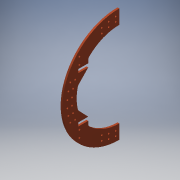
# Autodesk Inventor part: 16in inner coil
Saved by Autodesk Inventor 2016 (Build 200138000, 138)
## iProperties
Created: 2016-01-31
Part Number: 16in inner coil
Material: Copper
Document SubType Name: Modeling
Designer: Scott
Density: 8.94 g/cm^3
Appearance: Copper - Satin
Author: Scott
Autodesk Inventor part; units mm, degrees
ref_plane "YZ Plane" through (0, 0, 0) normal (1, 0, 0) x (0, 1, 0)
ref_plane "XZ Plane" through (0, 0, 0) normal (0, 1, 0) x (-1, 0, 0)
ref_plane "XY Plane" through (0, 0, 0) normal (0, 0, 1) x (1, 0, 0)
sketch "Sketch1" plane through (0, 0, 0) normal (1, 0, 0) x (0, 1, 0)
  arc A0 (203.2, 0) -> (-203.2, 0) centre (0, 0) ccw
  arc A1 (152.4, 0) -> (-152.4, 0) centre (0, 0) ccw
  arc A2 (185.42, 0) -> (-185.42, 0) centre (0, 0) ccw
  line L0 (0, 0) -> (152.4, 0) construction
  line L1 (0, 0) -> (220.2471, 220.2471) construction
  line L2 (0, 0) -> (-217.8171, 217.8171) construction
  line L3 (0, 0) -> (-152.4, 0) construction
  line L4 (203.2, 0) -> (418.8667, 0) construction
  line L5 (152.4, 0) -> (-185.42, 0)
  line L6 (-203.2, 0) -> (-272.3039, 0)
  line L7 (-185.42, 0) -> (-203.2, 0)
  line L8 (-152.4, 0) -> (-203.2, 0)
  line L9 (152.4, 0) -> (203.2, 0)
  arc A3 (168.91, 0) -> (-168.91, 0) centre (0, 0) ccw
  point P0 (181.5133, 37.8617)
  point P1 (184.9846, 12.7)
  point P2 (164.6231, 37.8128)
  point P3 (168.4319, 12.7)
  point P4 (174.6359, 62.3129)
  point P5 (157.0918, 62.0706)
  point P6 (37.8617, 181.5133)
  point P7 (12.7, 184.9846)
  point P8 (37.8128, 164.6231)
  point P9 (12.7, 168.4319)
  point P10 (62.3129, 174.6359)
  point P11 (62.0706, 157.0918)
  point P12 (-62.3129, 174.6359)
  point P13 (-37.8617, 181.5133)
  point P14 (-62.0706, 157.0918)
  point P15 (-37.8128, 164.6231)
  point P16 (-12.7, 168.4319)
  point P17 (-12.7, 184.9846)
  point P18 (-157.0918, 62.0706)
  point P19 (-174.6359, 62.3129)
  point P20 (-181.5133, 37.8617)
  point P21 (-164.6231, 37.8128)
  point P22 (-168.4319, 12.7)
  point P23 (-184.9846, 12.7)
  dimension "d0" = 406.4
  dimension "d2" = 304.8
  dimension "d3" = 370.84
  dimension "d5" = 50.8
  dimension "d6" = 25.4
  dimension "d7" = 25.4
  dimension "d8" = 12.7
  dimension "d9" = 12.7
  dimension "d10" = 25.4
  dimension "d11" = 25.4
  dimension "d12" = 45
  dimension "d13" = 45
  constraints: 20 end point, 16 point on circle, 12 symmetric about line, 4 centre point, 4 coincident, 3 horizontal, 3 point on line, 1 collinear
  measures "d0" diameter of A0
  measures "d2" diameter of A1
  measures "d3" diameter of A2
  measures "d5" radial gap between concentric circles of A1 A0
  measures "d6" distance of point (184.985, 12.7) point (181.513, 37.862)
  measures "d7" distance of point (168.432, 12.7) point (164.623, 37.813)
  measures "d8" distance from line of L0 point (184.985, 12.7)
  measures "d9" distance from line of L0 point (168.432, 12.7)
  measures "d10" distance of point (181.513, 37.862) point (174.636, 62.313)
  measures "d11" distance of point (164.623, 37.813) point (157.092, 62.071)
  measures "d12" angle of L3 L2
  measures "d13" angle of L0 L1
extrude "Extrusion1" add sketch "Sketch1" along normal blind 6.35 contours L9 A2 L7 A0 | L9 A3 L5 A2 | L9 A1 L5 A3
hole "Hole1" at (0, 181.5133, 37.8617) at (0, 184.9846, 12.7) at (0, 164.6231, 37.8128) at (0, 168.4319, 12.7) at (0, 174.6359, 62.3129) at (0, 157.0918, 62.0706) at (0, 62.3129, 174.6359) at (0, 37.8617, 181.5133) at (0, 62.0706, 157.0918) at (0, 37.8128, 164.6231) at (0, 12.7, 168.4319) at (0, 12.7, 184.9846) at (0, -62.0706, 157.0918) at (0, -62.3129, 174.6359) at (0, -37.8617, 181.5133) at (0, -37.8128, 164.6231) at (0, -12.7, 168.4319) at (0, -12.7, 184.9846) at (0, -184.9846, 12.7) at (0, -168.4319, 12.7) at (0, -181.5133, 37.8617) at (0, -164.6231, 37.8128) at (0, -174.6359, 62.3129) at (0, -157.0918, 62.0706) direction (1, 0, 0) diameter 6.604 end through all
sketch "Sketch4" plane through (0, 0, 0) normal (-1, 0, 0) x (0, 0, 1)
  line L0 (127, 92.2547) -> (157.48, 92.2547) projected
  line L1 (157.48, 150.1234) -> (157.48, 92.2547) projected
  line L2 (143.2518, 198.5102) -> (157.48, 150.1234) projected
  arc A0 (143.2518, 198.5102) -> (131.3752, 213.4606) centre (118.8834, 191.3446) ccw projected
  line L3 (127, 215.9318) -> (131.3752, 213.4606) projected
  line L4 (127, 92.2547) -> (127, 215.9318) projected
  circle A1 centre (142.24, 125.6507) radius 3.302 projected
  circle A2 centre (142.24, 100.2507) radius 3.302 projected
  circle A3 centre (142.24, -100.2507) radius 3.302 projected
  circle A4 centre (-142.24, -100.2507) radius 3.302 projected
  circle A5 centre (-142.24, -125.6507) radius 3.302 projected
  circle A6 centre (142.24, -125.6507) radius 3.302 projected
  line L5 (114.3, -183.162) -> (127, -183.162) projected
  line L6 (127, -183.162) -> (163.2323, -141.3083) projected
  arc A7 (163.2323, -141.3083) -> (215.9, 0) centre (0, 0) ccw projected
  line L7 (152.4, 0) -> (215.9, 0) projected
  arc A8 (-152.4, 0) -> (152.4, 0) centre (0, 0) ccw projected
  line L8 (-215.9, 0) -> (-152.4, 0) projected
  arc A9 (-215.9, 0) -> (-163.2323, -141.3083) centre (0, 0) ccw projected
  line L9 (-163.2323, -141.3083) -> (-127, -183.162) projected
  line L10 (-127, -183.162) -> (-114.3, -183.162) projected
  line L11 (-114.3, -183.162) -> (-114.3, -195.862) projected
  line L12 (-114.3, -195.862) -> (-46.5518, -210.8216) projected
  arc A10 (-46.5518, -210.8216) -> (46.5518, -210.8216) centre (0, 0) ccw projected
  line L13 (46.5518, -210.8216) -> (114.3, -195.862) projected
  line L14 (114.3, -195.862) -> (114.3, -183.162) projected
  circle A11 centre (174.6359, -62.3129) radius 3.302 projected
  circle A12 centre (181.5133, -37.8617) radius 3.302 projected
  circle A13 centre (184.9846, -12.7) radius 3.302 projected
  circle A14 centre (12.7, -168.4319) radius 3.302 projected
  circle A15 centre (37.8617, -181.5133) radius 3.302 projected
  circle A16 centre (62.0706, -157.0918) radius 3.302 projected
  circle A17 centre (-12.7, -168.4319) radius 3.302 projected
  circle A18 centre (-62.0706, -157.0918) radius 3.302 projected
  circle A19 centre (-62.3129, -174.6359) radius 3.302 projected
  circle A20 centre (-174.6359, -62.3129) radius 3.302 projected
  circle A21 centre (-164.6231, -37.8128) radius 3.302 projected
  circle A22 centre (-181.5133, -37.8617) radius 3.302 projected
  circle A23 centre (-184.9846, -12.7) radius 3.302 projected
  circle A24 centre (-168.4319, -12.7) radius 3.302 projected
  circle A25 centre (-157.0918, -62.0706) radius 3.302 projected
  circle A26 centre (-37.8617, -181.5133) radius 3.302 projected
  circle A27 centre (-37.8128, -164.6231) radius 3.302 projected
  circle A28 centre (-12.7, -184.9846) radius 3.302 projected
  circle A29 centre (62.3129, -174.6359) radius 3.302 projected
  circle A30 centre (37.8128, -164.6231) radius 3.302 projected
  circle A31 centre (12.7, -184.9846) radius 3.302 projected
  circle A32 centre (168.4319, -12.7) radius 3.302 projected
  circle A33 centre (164.6231, -37.8128) radius 3.302 projected
  circle A34 centre (157.0918, -62.0706) radius 3.302 projected
  point P0 (0, 0)
  constraints: 4 coincident
hole "Hole4" at (0, -125.6507, 142.24) at (0, -100.2507, 142.24) at (0, 100.2507, 142.24) at (0, 125.6507, 142.24) direction (1, 0, 0) diameter 6.604 end through all
sketch "Sketch5" plane through (0, 0, 0) normal (-1, 0, 0) x (0, 0, 1)
  line L0 (-145.9119, -88.9) -> (-106.6761, -88.9)
  line L1 (-106.6761, -88.9) -> (-106.6761, -76.2)
  line L2 (-106.6761, -76.2) -> (-145.9119, -76.2)
  line L3 (-145.9119, -76.2) -> (-145.9119, -88.9)
  line L4 (145.9119, -88.9) -> (99.5479, -88.9)
  line L5 (99.5479, -88.9) -> (99.5479, -76.2)
  line L6 (99.5479, -76.2) -> (145.9119, -76.2)
  line L7 (145.9119, -76.2) -> (145.9119, -88.9)
  line L8 (145.9119, 88.9) -> (145.9119, 76.2) projected
  line L9 (145.9119, 76.2) -> (108.0536, 76.2)
  line L10 (108.0536, 76.2) -> (108.0536, 88.9)
  line L11 (108.0536, 88.9) -> (145.9119, 88.9)
  line L12 (145.9119, 88.9) -> (145.9119, 76.2)
  point P0 (0, 0)
  constraints: 24 end point, 6 parallel, 3 horizontal, 3 perpendicular, 1 point on line
extrude "Extrusion3" cut sketch "Sketch5" against normal blind 25.4 contours L4 L5 L6 L7 | L8 L9 L10 L11
sketch "Sketch6" plane through (6.35, 0, 0) normal (1, 0, 0) x (0, 0, -1)
  circle A0 centre (-157.0918, 62.0706) radius 3.302 projected
  circle A1 centre (-164.6231, 37.8128) radius 3.302 projected
  circle A2 centre (-168.4319, 12.7) radius 3.302 projected
  circle A3 centre (-12.7, 184.9846) radius 3.302 projected
  circle A4 centre (-37.8128, 164.6231) radius 3.302 projected
  circle A5 centre (-62.3129, 174.6359) radius 3.302 projected
  circle A6 centre (12.7, 184.9846) radius 3.302 projected
  circle A7 centre (37.8128, 164.6231) radius 3.302 projected
  circle A8 centre (37.8617, 181.5133) radius 3.302 projected
  circle A9 centre (157.0918, 62.0706) radius 3.302 projected
  circle A10 centre (168.4319, 12.7) radius 3.302 projected
  circle A11 centre (184.9846, 12.7) radius 3.302 projected
  circle A12 centre (181.5133, 37.8617) radius 3.302 projected
  circle A13 centre (164.6231, 37.8128) radius 3.302 projected
  circle A14 centre (174.6359, 62.3129) radius 3.302 projected
  circle A15 centre (62.3129, 174.6359) radius 3.302 projected
  circle A16 centre (62.0706, 157.0918) radius 3.302 projected
  circle A17 centre (12.7, 168.4319) radius 3.302 projected
  circle A18 centre (-62.0706, 157.0918) radius 3.302 projected
  circle A19 centre (-37.8617, 181.5133) radius 3.302 projected
  circle A20 centre (-12.7, 168.4319) radius 3.302 projected
  circle A21 centre (-184.9846, 12.7) radius 3.302 projected
  circle A22 centre (-181.5133, 37.8617) radius 3.302 projected
  circle A23 centre (-174.6359, 62.3129) radius 3.302 projected
  line L0 (-123.8289, 76.2) -> (-145.9119, 76.2) projected
  line L1 (-145.9119, 76.2) -> (-145.9119, 88.9) projected
  line L2 (-145.9119, 88.9) -> (-123.7843, 88.9) projected
  arc A24 (123.7843, 88.9) -> (-123.7843, 88.9) centre (0, 0) ccw projected
  line L3 (123.7843, 88.9) -> (145.9119, 88.9) projected
  line L4 (145.9119, 88.9) -> (145.9119, 76.2) projected
  line L5 (145.9119, 76.2) -> (123.825, 76.2) projected
  line L6 (123.825, 76.2) -> (147.5607, 38.1) projected
  arc A25 (152.4, 0) -> (147.5607, 38.1) centre (0, 0) ccw projected
  line L7 (215.9, 0) -> (152.4, 0) projected
  arc A26 (215.9, 0) -> (163.2323, 141.3083) centre (0, 0) ccw projected
  line L8 (163.2323, 141.3083) -> (127, 183.162) projected
  line L9 (127, 183.162) -> (114.3, 183.162) projected
  line L10 (114.3, 183.162) -> (114.3, 195.862) projected
  line L11 (114.3, 195.862) -> (46.5518, 210.8216) projected
  arc A27 (46.5518, 210.8216) -> (-46.5518, 210.8216) centre (0, 0) ccw projected
  line L12 (-46.5518, 210.8216) -> (-114.3, 195.862) projected
  line L13 (-114.3, 195.862) -> (-114.3, 183.162) projected
  line L14 (-114.3, 183.162) -> (-127, 183.162) projected
  line L15 (-127, 183.162) -> (-163.2323, 141.3083) projected
  arc A28 (-163.2323, 141.3083) -> (-215.9, 0) centre (0, 0) ccw projected
  line L16 (-152.4, 0) -> (-215.9, 0) projected
  arc A29 (-147.5607, 38.1) -> (-152.4, 0) centre (0, 0) ccw projected
  line L17 (-147.5607, 38.1) -> (-123.8289, 76.2) projected
  circle A30 centre (-142.24, 125.6507) radius 3.302 projected
  circle A31 centre (142.24, 125.6507) radius 3.302 projected
  circle A32 centre (142.24, 100.2507) radius 3.302 projected
  circle A33 centre (-142.24, 100.2507) radius 3.302 projected
  circle A34 centre (157.0918, -62.0706) radius 3.302 projected
  circle A35 centre (164.6231, -37.8128) radius 3.302 projected
  circle A36 centre (168.4319, -12.7) radius 3.302 projected
  circle A37 centre (12.7, -184.9846) radius 3.302 projected
  circle A38 centre (37.8128, -164.6231) radius 3.302 projected
  circle A39 centre (62.3129, -174.6359) radius 3.302 projected
  circle A40 centre (-12.7, -184.9846) radius 3.302 projected
  circle A41 centre (-37.8128, -164.6231) radius 3.302 projected
  circle A42 centre (-37.8617, -181.5133) radius 3.302 projected
  circle A43 centre (-157.0918, -62.0706) radius 3.302 projected
  circle A44 centre (-168.4319, -12.7) radius 3.302 projected
  circle A45 centre (-184.9846, -12.7) radius 3.302 projected
  circle A46 centre (-181.5133, -37.8617) radius 3.302 projected
  circle A47 centre (-164.6231, -37.8128) radius 3.302 projected
  circle A48 centre (-174.6359, -62.3129) radius 3.302 projected
  circle A49 centre (-62.3129, -174.6359) radius 3.302 projected
  circle A50 centre (-62.0706, -157.0918) radius 3.302 projected
  circle A51 centre (-12.7, -168.4319) radius 3.302 projected
  circle A52 centre (62.0706, -157.0918) radius 3.302 projected
  circle A53 centre (37.8617, -181.5133) radius 3.302 projected
  circle A54 centre (12.7, -168.4319) radius 3.302 projected
  circle A55 centre (184.9846, -12.7) radius 3.302 projected
  circle A56 centre (181.5133, -37.8617) radius 3.302 projected
  circle A57 centre (174.6359, -62.3129) radius 3.302 projected
  line L18 (123.8289, -76.2) -> (145.9119, -76.2) projected
  line L19 (145.9119, -76.2) -> (145.9119, -88.9) projected
  line L20 (145.9119, -88.9) -> (123.7843, -88.9) projected
  arc A58 (-123.7843, -88.9) -> (123.7843, -88.9) centre (0, 0) ccw projected
  line L21 (-123.7843, -88.9) -> (-145.9119, -88.9) projected
  line L22 (-145.9119, -88.9) -> (-145.9119, -76.2) projected
  line L23 (-145.9119, -76.2) -> (-123.825, -76.2) projected
  line L24 (-123.825, -76.2) -> (-147.5607, -38.1) projected
  arc A59 (-152.4, 0) -> (-147.5607, -38.1) centre (0, 0) ccw projected
  line L25 (-215.9, 0) -> (-152.4, 0) projected
  arc A60 (-215.9, 0) -> (-163.2323, -141.3083) centre (0, 0) ccw projected
  line L26 (-163.2323, -141.3083) -> (-127, -183.162) projected
  line L27 (-127, -183.162) -> (-114.3, -183.162) projected
  line L28 (-114.3, -183.162) -> (-114.3, -195.862) projected
  line L29 (-114.3, -195.862) -> (-46.5518, -210.8216) projected
  arc A61 (-46.5518, -210.8216) -> (46.5518, -210.8216) centre (0, 0) ccw projected
  line L30 (46.5518, -210.8216) -> (114.3, -195.862) projected
  line L31 (114.3, -195.862) -> (114.3, -183.162) projected
  line L32 (114.3, -183.162) -> (127, -183.162) projected
  line L33 (127, -183.162) -> (163.2323, -141.3083) projected
  arc A62 (163.2323, -141.3083) -> (215.9, 0) centre (0, 0) ccw projected
  line L34 (152.4, 0) -> (215.9, 0) projected
  arc A63 (147.5607, -38.1) -> (152.4, 0) centre (0, 0) ccw projected
  line L35 (147.5607, -38.1) -> (123.8289, -76.2) projected
  circle A64 centre (142.24, -125.6507) radius 3.302 projected
  circle A65 centre (-142.24, -125.6507) radius 3.302 projected
  circle A66 centre (-142.24, -100.2507) radius 3.302 projected
  circle A67 centre (142.24, -100.2507) radius 3.302 projected
  arc A68 (-131.9823, 76.2) -> (-131.9823, -76.2) centre (0, 0) ccw projected
extrude "Extrusion4" add sketch "Sketch6" against normal blind 6.35 contours L17 A68 L0 | L24 L23 A68
sketch "Sketch7" plane through (6.35, 0, 0) normal (1, 0, 0) x (0, 0, -1)
  arc A0 (152.4, 0) -> (148.406, 34.6616) centre (0, 0) ccw projected
  line L0 (215.9, 0) -> (152.4, 0) projected
  arc A1 (215.9, 0) -> (163.2323, 141.3083) centre (0, 0) ccw projected
  line L1 (163.2323, 141.3083) -> (127, 183.162) projected
  line L2 (127, 183.162) -> (114.3, 183.162) projected
  line L3 (114.3, 183.162) -> (114.3, 195.862) projected
  line L4 (114.3, 195.862) -> (46.5518, 210.8216) projected
  arc A2 (46.5518, 210.8216) -> (-46.5518, 210.8216) centre (0, 0) ccw projected
  line L5 (-46.5518, 210.8216) -> (-114.3, 195.862) projected
  line L6 (-114.3, 195.862) -> (-114.3, 183.162) projected
  line L7 (-114.3, 183.162) -> (-127, 183.162) projected
  line L8 (-127, 183.162) -> (-163.2323, 141.3083) projected
  arc A3 (-163.2323, 141.3083) -> (-215.9, 0) centre (0, 0) ccw projected
  line L9 (-152.4, 0) -> (-215.9, 0) projected
  arc A4 (-148.406, 34.6616) -> (-152.4, 0) centre (0, 0) ccw projected
  arc A5 (-145.2178, 40.5502) -> (-148.406, 34.6616) centre (-136.0388, 31.7731) ccw projected
  line L10 (-145.2178, 40.5502) -> (-111.1289, 76.2) projected
  line L11 (-111.1289, 76.2) -> (-145.9119, 76.2) projected
  line L12 (-145.9119, 76.2) -> (-145.9119, 88.9) projected
  line L13 (-145.9119, 88.9) -> (-111.0843, 88.9) projected
  line L14 (-111.0843, 88.9) -> (-111.0843, 99.1797) projected
  arc A6 (-107.3283, 108.1961) -> (-111.0843, 99.1797) centre (-98.3843, 99.1797) ccw projected
  arc A7 (107.3283, 108.1961) -> (-107.3283, 108.1961) centre (0, 0) ccw projected
  arc A8 (111.0843, 99.1797) -> (107.3283, 108.1961) centre (98.3843, 99.1797) ccw projected
  line L15 (111.0843, 88.9) -> (111.0843, 99.1797) projected
  line L16 (111.0843, 88.9) -> (145.9119, 88.9) projected
  line L17 (145.9119, 88.9) -> (145.9119, 76.2) projected
  line L18 (145.9119, 76.2) -> (111.1289, 76.2) projected
  line L19 (145.2178, 40.5502) -> (111.1289, 76.2) projected
  arc A9 (148.406, 34.6616) -> (145.2178, 40.5502) centre (136.0388, 31.7731) ccw projected
  circle A10 centre (-157.0918, 62.0706) radius 3.302 projected
  circle A11 centre (-164.6231, 37.8128) radius 3.302 projected
  circle A12 centre (-168.4319, 12.7) radius 3.302 projected
  circle A13 centre (-12.7, 184.9846) radius 3.302 projected
  circle A14 centre (-37.8128, 164.6231) radius 3.302 projected
  circle A15 centre (-62.3129, 174.6359) radius 3.302 projected
  circle A16 centre (12.7, 184.9846) radius 3.302 projected
  circle A17 centre (37.8128, 164.6231) radius 3.302 projected
  circle A18 centre (37.8617, 181.5133) radius 3.302 projected
  circle A19 centre (157.0918, 62.0706) radius 3.302 projected
  circle A20 centre (168.4319, 12.7) radius 3.302 projected
  circle A21 centre (184.9846, 12.7) radius 3.302 projected
  circle A22 centre (181.5133, 37.8617) radius 3.302 projected
  circle A23 centre (164.6231, 37.8128) radius 3.302 projected
  circle A24 centre (174.6359, 62.3129) radius 3.302 projected
  circle A25 centre (62.3129, 174.6359) radius 3.302 projected
  circle A26 centre (62.0706, 157.0918) radius 3.302 projected
  circle A27 centre (12.7, 168.4319) radius 3.302 projected
  circle A28 centre (-62.0706, 157.0918) radius 3.302 projected
  circle A29 centre (-37.8617, 181.5133) radius 3.302 projected
  circle A30 centre (-12.7, 168.4319) radius 3.302 projected
  circle A31 centre (-184.9846, 12.7) radius 3.302 projected
  circle A32 centre (-181.5133, 37.8617) radius 3.302 projected
  circle A33 centre (-174.6359, 62.3129) radius 3.302 projected
  circle A34 centre (-142.24, 125.6507) radius 3.302 projected
  circle A35 centre (142.24, 125.6507) radius 3.302 projected
  circle A36 centre (142.24, 100.2507) radius 3.302 projected
  circle A37 centre (-142.24, 100.2507) radius 3.302 projected
  arc A38 (-152.4, 0) -> (-148.406, -34.6616) centre (0, 0) ccw projected
  line L20 (-215.9, 0) -> (-152.4, 0) projected
  arc A39 (-215.9, 0) -> (-163.2323, -141.3083) centre (0, 0) ccw projected
  line L21 (-163.2323, -141.3083) -> (-127, -183.162) projected
  line L22 (-127, -183.162) -> (-114.3, -183.162) projected
  line L23 (-114.3, -183.162) -> (-114.3, -195.862) projected
  line L24 (-114.3, -195.862) -> (-46.5518, -210.8216) projected
  arc A40 (-46.5518, -210.8216) -> (46.5518, -210.8216) centre (0, 0) ccw projected
  line L25 (46.5518, -210.8216) -> (114.3, -195.862) projected
  line L26 (114.3, -195.862) -> (114.3, -183.162) projected
  line L27 (114.3, -183.162) -> (127, -183.162) projected
  line L28 (127, -183.162) -> (163.2323, -141.3083) projected
  arc A41 (163.2323, -141.3083) -> (215.9, 0) centre (0, 0) ccw projected
  line L29 (152.4, 0) -> (215.9, 0) projected
  arc A42 (148.406, -34.6616) -> (152.4, 0) centre (0, 0) ccw projected
  arc A43 (145.2178, -40.5502) -> (148.406, -34.6616) centre (136.0388, -31.7731) ccw projected
  line L30 (145.2178, -40.5502) -> (111.1289, -76.2) projected
  line L31 (111.1289, -76.2) -> (145.9119, -76.2) projected
  line L32 (145.9119, -76.2) -> (145.9119, -88.9) projected
  line L33 (145.9119, -88.9) -> (111.0843, -88.9) projected
  line L34 (111.0843, -88.9) -> (111.0843, -99.1797) projected
  arc A44 (107.3283, -108.1961) -> (111.0843, -99.1797) centre (98.3843, -99.1797) ccw projected
  arc A45 (-107.3283, -108.1961) -> (107.3283, -108.1961) centre (0, 0) ccw projected
  arc A46 (-111.0843, -99.1797) -> (-107.3283, -108.1961) centre (-98.3843, -99.1797) ccw projected
  line L35 (-111.0843, -88.9) -> (-111.0843, -99.1797) projected
  line L36 (-111.0843, -88.9) -> (-145.9119, -88.9) projected
  line L37 (-145.9119, -88.9) -> (-145.9119, -76.2) projected
  line L38 (-145.9119, -76.2) -> (-111.1289, -76.2) projected
  line L39 (-145.2178, -40.5502) -> (-111.1289, -76.2) projected
  arc A47 (-148.406, -34.6616) -> (-145.2178, -40.5502) centre (-136.0388, -31.7731) ccw projected
  circle A48 centre (157.0918, -62.0706) radius 3.302 projected
  circle A49 centre (164.6231, -37.8128) radius 3.302 projected
  circle A50 centre (168.4319, -12.7) radius 3.302 projected
  circle A51 centre (12.7, -184.9846) radius 3.302 projected
  circle A52 centre (37.8128, -164.6231) radius 3.302 projected
  circle A53 centre (62.3129, -174.6359) radius 3.302 projected
  circle A54 centre (-12.7, -184.9846) radius 3.302 projected
  circle A55 centre (-37.8128, -164.6231) radius 3.302 projected
  circle A56 centre (-37.8617, -181.5133) radius 3.302 projected
  circle A57 centre (-157.0918, -62.0706) radius 3.302 projected
  circle A58 centre (-168.4319, -12.7) radius 3.302 projected
  circle A59 centre (-184.9846, -12.7) radius 3.302 projected
  circle A60 centre (-181.5133, -37.8617) radius 3.302 projected
  circle A61 centre (-164.6231, -37.8128) radius 3.302 projected
  circle A62 centre (-174.6359, -62.3129) radius 3.302 projected
  circle A63 centre (-62.3129, -174.6359) radius 3.302 projected
  circle A64 centre (-62.0706, -157.0918) radius 3.302 projected
  circle A65 centre (-12.7, -168.4319) radius 3.302 projected
  circle A66 centre (62.0706, -157.0918) radius 3.302 projected
  circle A67 centre (37.8617, -181.5133) radius 3.302 projected
  circle A68 centre (12.7, -168.4319) radius 3.302 projected
  circle A69 centre (184.9846, -12.7) radius 3.302 projected
  circle A70 centre (181.5133, -37.8617) radius 3.302 projected
  circle A71 centre (174.6359, -62.3129) radius 3.302 projected
  circle A72 centre (142.24, -125.6507) radius 3.302 projected
  circle A73 centre (-142.24, -125.6507) radius 3.302 projected
  circle A74 centre (-142.24, -100.2507) radius 3.302 projected
  circle A75 centre (142.24, -100.2507) radius 3.302 projected
  line L40 (0, -259.08) -> (0, 43.18)
  line L41 (0, -215.9) -> (0, 215.9)
  arc A76 (152.4, 0) -> (148.406, 34.6616) centre (0, 0) ccw projected
  line L42 (215.9, 0) -> (152.4, 0) projected
  arc A77 (215.9, 0) -> (163.2323, 141.3083) centre (0, 0) ccw projected
  line L43 (163.2323, 141.3083) -> (127, 183.162) projected
  line L44 (127, 183.162) -> (114.3, 183.162) projected
  line L45 (114.3, 183.162) -> (114.3, 195.862) projected
  line L46 (114.3, 195.862) -> (46.5518, 210.8216) projected
  arc A78 (46.5518, 210.8216) -> (-46.5518, 210.8216) centre (0, 0) ccw projected
  line L47 (-46.5518, 210.8216) -> (-114.3, 195.862) projected
  line L48 (-114.3, 195.862) -> (-114.3, 183.162) projected
  line L49 (-114.3, 183.162) -> (-127, 183.162) projected
  line L50 (-127, 183.162) -> (-163.2323, 141.3083) projected
  arc A79 (-163.2323, 141.3083) -> (-215.9, 0) centre (0, 0) ccw projected
  line L51 (-152.4, 0) -> (-215.9, 0) projected
  arc A80 (-148.406, 34.6616) -> (-152.4, 0) centre (0, 0) ccw projected
  arc A81 (-145.2178, 40.5502) -> (-148.406, 34.6616) centre (-136.0388, 31.7731) ccw projected
  line L52 (-145.2178, 40.5502) -> (-111.1289, 76.2) projected
  line L53 (-111.1289, 76.2) -> (-145.9119, 76.2) projected
  line L54 (-145.9119, 76.2) -> (-145.9119, 88.9) projected
  line L55 (-145.9119, 88.9) -> (-111.0843, 88.9) projected
  line L56 (-111.0843, 88.9) -> (-111.0843, 99.1797) projected
  arc A82 (-107.3283, 108.1961) -> (-111.0843, 99.1797) centre (-98.3843, 99.1797) ccw projected
  arc A83 (107.3283, 108.1961) -> (-107.3283, 108.1961) centre (0, 0) ccw projected
  arc A84 (111.0843, 99.1797) -> (107.3283, 108.1961) centre (98.3843, 99.1797) ccw projected
  line L57 (111.0843, 88.9) -> (111.0843, 99.1797) projected
  line L58 (111.0843, 88.9) -> (145.9119, 88.9) projected
  line L59 (145.9119, 88.9) -> (145.9119, 76.2) projected
  line L60 (145.9119, 76.2) -> (111.1289, 76.2) projected
  line L61 (145.2178, 40.5502) -> (111.1289, 76.2) projected
  arc A85 (148.406, 34.6616) -> (145.2178, 40.5502) centre (136.0388, 31.7731) ccw projected
  circle A86 centre (-157.0918, 62.0706) radius 3.302 projected
  circle A87 centre (-164.6231, 37.8128) radius 3.302 projected
  circle A88 centre (-168.4319, 12.7) radius 3.302 projected
  circle A89 centre (-12.7, 184.9846) radius 3.302 projected
  circle A90 centre (-37.8128, 164.6231) radius 3.302 projected
  circle A91 centre (-62.3129, 174.6359) radius 3.302 projected
  circle A92 centre (12.7, 184.9846) radius 3.302 projected
  circle A93 centre (37.8128, 164.6231) radius 3.302 projected
  circle A94 centre (37.8617, 181.5133) radius 3.302 projected
  circle A95 centre (157.0918, 62.0706) radius 3.302 projected
  circle A96 centre (168.4319, 12.7) radius 3.302 projected
  circle A97 centre (184.9846, 12.7) radius 3.302 projected
  circle A98 centre (181.5133, 37.8617) radius 3.302 projected
  circle A99 centre (164.6231, 37.8128) radius 3.302 projected
  circle A100 centre (174.6359, 62.3129) radius 3.302 projected
  circle A101 centre (62.3129, 174.6359) radius 3.302 projected
  circle A102 centre (62.0706, 157.0918) radius 3.302 projected
  circle A103 centre (12.7, 168.4319) radius 3.302 projected
  circle A104 centre (-62.0706, 157.0918) radius 3.302 projected
  circle A105 centre (-37.8617, 181.5133) radius 3.302 projected
  circle A106 centre (-12.7, 168.4319) radius 3.302 projected
  circle A107 centre (-184.9846, 12.7) radius 3.302 projected
  circle A108 centre (-181.5133, 37.8617) radius 3.302 projected
  circle A109 centre (-174.6359, 62.3129) radius 3.302 projected
  circle A110 centre (-142.24, 125.6507) radius 3.302 projected
  circle A111 centre (142.24, 125.6507) radius 3.302 projected
  circle A112 centre (142.24, 100.2507) radius 3.302 projected
  circle A113 centre (-142.24, 100.2507) radius 3.302 projected
  arc A114 (0, 152.4) -> (-123.7843, 88.9) centre (0, 0) ccw projected
  line L62 (-147.5607, 38.1) -> (-123.8289, 76.2) projected
  line L63 (-123.825, -76.2) -> (-147.5607, -38.1) projected
  arc A115 (-147.5607, 38.1) -> (-147.5607, -38.1) centre (0, 0) ccw projected
  arc A116 (-123.7843, -88.9) -> (0, -152.4) centre (0, 0) ccw projected
  constraints: 4 end point, 2 point on circle, 1 point on line, 1 vertical, 2 other
extrude "Extrusion5" add sketch "Sketch7" against normal blind 6.35 contours A6 L14 L13 A114 | A116 L36 L35 A46 | L11 L10 A5 A115 L62 | L63 A115 A47 L39 L38
body "Solid1"
